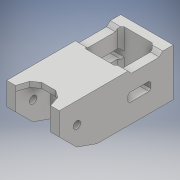
# Autodesk Inventor part: holder-GT2-x-carriage-V2-left
Saved by Autodesk Inventor 2018 (Build 220112000, 112)
## iProperties
Created: 2018-02-18
Part Number: holder-GT2-x-carriage-V2-left
Material: Generic
Document SubType Name: Modeling
Designer: Jurjen
Density: 1 g/cm^3
Appearance: Default
Author: Jurjen
Autodesk Inventor part; units mm, degrees
ref_plane "YZ Plane" through (0, 0, 0) normal (1, 0, 0) x (0, 1, 0)
ref_plane "XZ Plane" through (0, 0, 0) normal (0, 1, 0) x (-1, 0, 0)
ref_plane "XY Plane" through (0, 0, 0) normal (0, 0, 1) x (1, 0, 0)
sketch "Sketch1" plane through (0, 0, 0) normal (0, 0, 1) x (1, 0, 0)
  line L0 (-10, 10.95) -> (10, 10.95)
  line L1 (10, 10.95) -> (10, -10.95)
  line L2 (10, -10.95) -> (-10, -10.95)
  line L3 (-10, -10.95) -> (-10, 10.95)
  line L4 (-15, 15.95) -> (15, 15.95)
  line L5 (15, 15.95) -> (15, -29.05)
  line L6 (15, -29.05) -> (10, -29.05) construction
  line L7 (-15, -29.05) -> (-15, 15.95)
  line L8 (-15, -29.05) -> (-10, -29.05) construction
  line L9 (-10, -29.05) -> (-10, -49.05)
  line L10 (-10, -49.05) -> (-15, -49.05)
  line L11 (-15, -49.05) -> (-15, -29.05)
  line L12 (15, -29.05) -> (10, -29.05) construction
  line L13 (10, -29.05) -> (10, -49.05)
  line L14 (10, -49.05) -> (15, -49.05)
  line L15 (15, -49.05) -> (15, -29.05)
  line L16 (-10, -29.05) -> (-15, -29.05) construction
  line L17 (10, -29.05) -> (-10, -29.05)
  point P0 (0, 0)
  point P1 (0, 10.95)
  point P2 (10, 0)
  dimension "d8" = 0
  dimension "d0" = 20
  dimension "d1" = 21.9
  dimension "d2" = 5
  dimension "d3" = 5
  dimension "d4" = 5
  dimension "d5" = 18.1
  dimension "d6" = 20
  constraints: 36 end point, 10 parallel, 4 horizontal, 4 perpendicular, 3 vertical alignment, 2 horizontal alignment, 2 midpoint, 1 point on line
  measures "d0" distance between parallel lines of L1 L3
  measures "d1" distance of L2.end L0.start
  measures "d2" distance between parallel lines of L4 L0
  measures "d3" distance between parallel lines of L5 L1
  measures "d4" distance between parallel lines of L7 L3
  measures "d5" distance between parallel lines of L6 L2
  measures "d6" distance between parallel lines of L14 L6
extrude "Extrusion1" add sketch "Sketch1" along normal mid plane 27
sketch "Sketch3" plane through (-15, 15.95, 13.5) normal (0, 1, 0) x (1, 0, 0)
  circle A0 centre (15, 20) radius 2.6
  line L0 (0, 27) -> (30, 27) projected
  point P0 (15, 13.5)
  point P1 (15, 27)
  dimension "d9" = 5.2
  dimension "d10" = 7
  constraints: 1 centre point, 1 midpoint, 1 vertical alignment
  measures "d9" diameter of A0
  measures "d10" distance from line of L0 A0.centre
extrude "Extrusion2" cut sketch "Sketch3" against normal through all
sketch "Sketch4" plane through (-10, -29.05, 13.5) normal (0, -1, 0) x (1, 0, 0)
  circle A0 centre (10, -20) radius 2.6 projected
  line L0 (14.15, -22.5524) -> (14.15, -17.4476)
  line L1 (14.15, -17.4476) -> (10, -15.35)
  line L2 (10, -15.35) -> (5.85, -17.4476)
  line L3 (5.85, -17.4476) -> (5.85, -22.5524)
  line L4 (5.85, -22.5524) -> (10, -24.65)
  line L5 (10, -24.65) -> (14.15, -22.5524)
  point P0 (10, -13.5)
  point P1 (14.15, -20)
  dimension "d13" = 9.3
  dimension "d14" = 8.3
  dimension "d15" = 8.3
  constraints: 12 end point, 4 parallel, 3 horizontal alignment, 2 vertical alignment, 1 midpoint, 1 vertical
  measures "d13" distance of L1.end L4.end
  measures "d14" distance between parallel lines of L3 L0
  measures "d15" distance between parallel lines of L4 L1
extrude "Extrusion3" cut sketch "Sketch4" against normal blind 14
sketch "Sketch5" plane through (0, 0, 13.5) normal (0, 0, 1) x (1, 0, 0)
  line L0 (10, -29.05) -> (10, -49.05) projected
  line L1 (-10, -29.05) -> (10, -29.05) projected
  line L2 (-10, -49.05) -> (-10, -29.05) projected
  line L3 (10, -29.05) -> (-10, -29.05)
  line L4 (-10, -29.05) -> (-10, -49.05)
  line L5 (-10, -49.05) -> (10, -49.05)
  line L6 (10, -49.05) -> (10, -29.05)
  point P0 (0, 0)
  constraints: 8 end point, 2 parallel, 1 horizontal, 1 perpendicular
extrude "Extrusion4" add sketch "Sketch5" against normal blind 3
sketch "Sketch6" plane through (15, -49.05, 13.5) normal (1, 0, 0) x (0, 0, -1)
  line L0 (27, 60) -> (27, 38.1) projected
  line L1 (11, 60) -> (16, 60)
  line L2 (16, 60) -> (16, 48)
  line L3 (16, 48) -> (11, 48)
  line L4 (11, 48) -> (11, 60)
  line L5 (17.4, 65) -> (22.6, 65) projected
  line L6 (0, 65) -> (27, 65) projected
  point P0 (13.5, 49.05)
  point P1 (20, 65)
  point P2 (20, 65)
  dimension "d20" = 5
  dimension "d21" = 12
  dimension "d32" = 4
  constraints: 8 end point, 2 parallel, 1 coincident, 1 horizontal, 1 horizontal alignment, 1 midpoint, 1 perpendicular, 1 point on line
  measures "d20" distance between parallel lines of L2 L4
  measures "d21" distance between parallel lines of L3 L1
  measures "d32" distance from line of point (20, 65) L2
extrude "Extrusion5" cut sketch "Sketch6" against normal blind 20 from surface at -25
sketch "Sketch7" plane through (-15, -49.05, 13.5) normal (-1, 0, 0) x (0, 0, 1)
  line L0 (0, 65) -> (-27, 65) projected
  line L1 (0, 0) -> (0, 65) projected
  line L2 (0, 0) -> (-27, 0) projected
  line L3 (-27, 65) -> (-27, 0) projected
  line L4 (-16, 52.1) -> (-11, 52.1)
  line L5 (-11, 52.1) -> (-11, 39.1)
  line L6 (-11, 39.1) -> (-16, 39.1)
  line L7 (-16, 39.1) -> (-16, 52.1)
  point P0 (-13.5, 49.05)
  point P1 (-27, 38.1)
  dimension "d25" = 5
  dimension "d26" = 13
  dimension "d62" = 1
  constraints: 8 end point, 2 parallel, 1 horizontal, 1 perpendicular
  measures "d25" distance between parallel lines of L5 L7
  measures "d26" distance between parallel lines of L6 L4
  measures "d62" distance from line of point (-27, 38.1) L6
extrude "Extrusion6" cut sketch "Sketch7" against normal blind 8 from surface at -25 contours L4 L5 L6 L7
chamfer "Chamfer1" distance 1 angle 45 8 edges at (12.5, 3.05, 2.5) (12.5, 3.05, -2.5) (-12.5, -1.05, 2.5) (-12.5, -1.05, -2.5) (12.5, -9.95, -2.5) (12.5, -9.95, 2.5) (-12.5, 10.95, 2.5) (-12.5, 10.95, -2.5)
sketch "Sketch8" plane through (15, -49.05, 13.5) normal (1, 0, 0) x (0, 0, -1)
  circle A0 centre (12, 10) radius 2.1
  line L0 (0, 0) -> (27, 0) projected
  point P0 (13.5, 49.05)
  dimension "d33" = 4.2
  dimension "d34" = 10
  dimension "d35" = 15
  constraints: 1 centre point
  measures "d33" diameter of A0
  measures "d34" distance from line of L0 A0.centre
  measures "d35" horizontal distance of L0.end A0.centre
extrude "Extrusion7" cut sketch "Sketch8" against normal through all
sketch "Sketch9" plane through (0, 0, 13.5) normal (0, 0, 1) x (1, 0, 0)
  line L0 (10, -29.05) -> (-10, -29.05) projected
  line L1 (10, -49.05) -> (10, -29.05) projected
  line L2 (10, -49.05) -> (-10, -49.05) projected
  line L3 (-10, -29.05) -> (-10, -49.05) projected
  line L4 (-10, -49.05) -> (-7, -40.05)
  line L5 (-7, -40.05) -> (7, -40.05)
  line L6 (10, -49.05) -> (10, -29.05) projected
  line L7 (7, -40.05) -> (10, -49.05)
  point P0 (0, 0)
  dimension "d38" = 9
  dimension "d39" = 3
  constraints: 6 end point, 1 equal length, 1 horizontal
  measures "d38" distance between parallel lines of L2 L5
  measures "d39" horizontal distance of L2.end L4.end
extrude "Extrusion8" cut sketch "Sketch9" against normal up to next contours L2 L4 L5 L7
chamfer "Chamfer2" distance 3 angle 45 2 edges at (-7, -40.05, 12) (7, -40.05, 12)
sketch "Sketch10" plane through (-10, -29.05, -13.5) normal (0, -1, 0) x (1, 0, 0)
  line L0 (20, 24) -> (0, 24) projected
  line L1 (0, 24) -> (0, 0) projected
  line L2 (20, 0) -> (0, 0) projected
  line L3 (10, 11.65) -> (14.15, 9.5524) projected
  line L4 (14.15, 9.5524) -> (14.15, 4.4476) projected
  line L5 (14.15, 4.4476) -> (10, 2.35) projected
  line L6 (10, 2.35) -> (5.85, 4.4476) projected
  line L7 (5.85, 4.4476) -> (5.85, 9.5524) projected
  line L8 (5.85, 9.5524) -> (10, 11.65) projected
  line L9 (20, 24) -> (0, 24) projected
  line L10 (0, 24) -> (4, 17.5)
  line L11 (4, 17.5) -> (16, 17.5)
  line L12 (16, 17.5) -> (20, 24)
  line L13 (20, 24) -> (20, 0) projected
  point P0 (10, 13.5)
  point P1 (10, 17.5)
  point P2 (10, 24)
  dimension "d45" = 6.5
  dimension "d46" = 12
  constraints: 6 end point, 2 midpoint, 1 parallel, 1 vertical alignment
  measures "d45" distance between parallel lines of L0 L11
  measures "d46" distance of L11.end L10.end
extrude "Extrusion9" cut sketch "Sketch10" against normal blind 10 contours L12 L11 L10 L0
chamfer "Chamfer3" distance 4 angle 45 2 edges at (6, -24.05, 4) (-6, -24.05, 4)
sketch "Sketch11" plane through (0, 0, -13.5) normal (0, 0, -1) x (-1, 0, 0)
  line L0 (8.0964, -29.05) -> (2, -29.05) projected
  line L1 (-6.5, -20.05) -> (6.5, -20.05)
  line L2 (6.5, -20.05) -> (6.5, -29.05)
  line L3 (6.5, -29.05) -> (-6.5, -29.05)
  line L4 (-6.5, -29.05) -> (-6.5, -20.05)
  line L5 (-10, -29.05) -> (10, -29.05) projected
  point P0 (0, 0)
  point P1 (0, -20.05)
  point P2 (0, -29.05)
  dimension "d52" = 13
  dimension "d53" = 9
  constraints: 8 end point, 2 midpoint, 2 parallel, 1 horizontal, 1 perpendicular, 1 point on line, 1 vertical alignment
  measures "d52" distance between parallel lines of L2 L4
  measures "d53" distance between parallel lines of L0 L1
extrude "Extrusion10" cut sketch "Sketch11" against normal blind 12
sketch "Sketch12" plane through (15, -49.05, 13.5) normal (1, 0, 0) x (0, 0, -1)
  line L0 (0, 0) -> (27, 0) projected
  line L1 (13, 0) -> (27, 14)
  line L2 (27, 65) -> (27, 0) projected
  line L3 (22.9, 9.9) -> (27, 21.5)
  point P0 (13.5, 49.05)
  dimension "d56" = 45
  dimension "d57" = 14
  dimension "d58" = 4.1
  dimension "d59" = 7.5
  constraints: 4 end point, 3 point on line, 1 vertical alignment
  measures "d56" angle of L1 L2
  measures "d57" distance of L0.end L1.end
  measures "d58" horizontal distance of L3.start L1.end
  measures "d59" distance of L1.end L3.end
extrude "Extrusion11" cut sketch "Sketch12" against normal through all
sketch "Sketch13" plane through (-15, -49.05, 13.5) normal (-1, 0, 0) x (0, 0, 1)
  line L0 (-22.9, 9.9) -> (-13, 0) projected
  line L1 (0, 0) -> (-13, 0) projected
  line L2 (0, 65) -> (0, 0) projected
  line L3 (-27, 65) -> (0, 65) projected
  line L4 (-27, 21.5) -> (-27, 65) projected
  line L5 (-27, 21.5) -> (-22.9, 9.9) projected
  circle A0 centre (-12, 10) radius 2.1 projected
  line L6 (0, 38.1) -> (0, 60) projected
  line L7 (0, 41.1) -> (-2, 41.1)
  line L8 (-2, 41.1) -> (-2, 57)
  line L9 (-2, 57) -> (0, 57)
  line L10 (-11, 59) -> (-11, 49) projected
  line L11 (-16, 49) -> (-16, 59) projected
  line L12 (-15, 60) -> (-16, 59) projected
  line L13 (-15, 60) -> (-12, 60) projected
  line L14 (-11, 59) -> (-12, 60) projected
  line L15 (-12, 48) -> (-11, 49) projected
  line L16 (-12, 48) -> (-15, 48) projected
  line L17 (-16, 49) -> (-15, 48) projected
  dimension "d9" = 5.2
  dimension "d63" = 2
  dimension "d75" = 3
  dimension "d76" = 3
  constraints: 6 end point, 2 perpendicular, 2 point on line, 1 horizontal
  measures "d63" distance between parallel lines of L6 L8
  measures "d75" distance from line of L6.end L9
  measures "d76" distance from line of L6.start L7
extrude "Extrusion12" cut sketch "Sketch13" against normal through all contours L7 L8 L9 L2
chamfer "Chamfer4" distance 2 angle 45 4 edges at (-12.5, -7.95, 13.5) (-12.5, 7.95, 13.5) (12.5, -7.95, 13.5) (12.5, 7.95, 13.5)
sketch "Sketch14" plane through (0, 0, 13.5) normal (0, 0, 1) x (1, 0, 0)
  line L0 (-10, 9.95) -> (-10, 10.95) projected
  line L1 (-10, 9.95) -> (-9, 10.95)
  line L2 (10, -0.05) -> (10, 9.95) projected
  line L3 (-10, 10.95) -> (10, 10.95) projected
  line L4 (10, 10.95) -> (9, 10.95)
  line L5 (10, 9.95) -> (10, 10.95)
  line L6 (9, 10.95) -> (10, 9.95)
  point P0 (0, 0)
  dimension "d69" = 45
  constraints: 8 end point, 3 horizontal alignment, 2 perpendicular, 1 point on line
  measures "d69" angle of L0 L1
extrude "Extrusion13" add sketch "Sketch14" against normal blind 4
chamfer "Chamfer5" distance 2 angle 45 5 edges at (-10, -10.95, 0) (10, -10.95, 0) (-10, 10.95, 5.5) (-10, 10.95, -7.5) (10, 10.95, -2)
equation "\"d4\" = d3"
body "Solid1"
